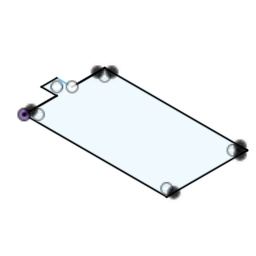
PCB+BOX+V2 (Autodesk Fusion 360 design; units mm, degrees)
Autodesk Fusion 360 part; units mm, degrees
sketch "PCB" plane through (0, 0, 0) normal (0, 0, 1) x (1, 0, 0)
  line L0 (0, 0) -> (92.87, 0)
  line L1 (92.87, 0) -> (92.87, 52.44)
  line L2 (92.87, 52.44) -> (0, 52.44)
  line L3 (0, 0) -> (0, 21.22)
  line L4 (0, 52.44) -> (0, 31.22)
  line L5 (0, 21.22) -> (-10, 21.22)
  line L6 (-10, 21.22) -> (-10, 31.22)
  line L7 (-10, 31.22) -> (0, 31.22)
  line L8 (0, 52.44) -> (0, 31.22)
  line L9 (0, 21.22) -> (0, 0)
  circle A0 centre (-5, 26.22) radius 2.5
  line L10 (0, 52.44) -> (4.6, 52.44)
  line L11 (0, 52.44) -> (0, 47.84)
  circle A1 centre (4.6, 47.84) radius 2
  line L12 (92.87, 52.44) -> (88.27, 52.44)
  line L13 (92.87, 52.44) -> (92.87, 47.84)
  circle A2 centre (88.27, 47.84) radius 2
  line L14 (92.87, 0) -> (92.87, 4.6)
  circle A3 centre (88.27, 4.6) radius 2
  line L15 (0, 0) -> (0, 4.6)
  circle A4 centre (4.6, 4.6) radius 2
  dimension "d8" = 92.87
  dimension "d9" = 52.44
  dimension "d10" = 21.22
  dimension "d11" = 21.22
  dimension "d12" = 10
  dimension "d13" = 5
  dimension "d14" = 4.6
  dimension "d15" = 4.6
  dimension "d16" = 4
  dimension "d17" = 4.6
  dimension "d18" = 4.6
  dimension "d19" = 4
  dimension "d20" = 4.6
  dimension "d21" = 4
  dimension "d22" = 4.6
  dimension "d23" = 4
  constraint horizontal L0
  constraint vertical L1
  constraint horizontal L2
  constraint vertical L8
  constraint coincident L0.start L3.start
  constraint coincident L3.end L8
  constraint horizontal L5
  constraint vertical L6
  constraint horizontal L7
  constraint collinear L8 L9
  constraint perpendicular L4 L10
  constraint perpendicular L2 L11
  constraint perpendicular L1 L12
  constraint perpendicular L12 L13
  constraint perpendicular L2 L14
  constraint perpendicular L0 L15
  measures "d8" distance of L0.start L0.end
  measures "d9" distance of L0.start L2.end
  measures "d10" distance of L0.start L3.end
  measures "d11" distance of L2.end L4.end
  measures "d12" distance of L3.end L5.end
  measures "d13" diameter of A0
  measures "d14" distance of L2.end L10.end
  measures "d15" distance of L2.end L11.end
  measures "d16" diameter of A1
  measures "d17" distance of L1.end L12.end
  measures "d18" distance of L1.end L13.end
  measures "d19" diameter of A2
  measures "d20" distance of L0.end L14.end
  measures "d21" diameter of A3
  measures "d22" distance of L0.start L15.end
  measures "d23" diameter of A4
extrude "Extrude1" add sketch "PCB" along normal blind 1.6 makes body 1
sketch "PCB BOX" plane through (0, 0, 0) normal (0, 0, 1) x (1, 0, 0)
  line L0 (-14.127, 62.44) -> (96.997, 62.44)
  line L1 (102.87, 56.567) -> (102.87, -4.127)
  line L2 (96.997, -10) -> (-14.127, -10)
  line L3 (-20, -4.127) -> (-20, 56.567)
  line L4 (92.87, 52.44) -> (0, 52.44)
  line L5 (92.87, 0) -> (92.87, 52.44)
  line L6 (0, 0) -> (92.87, 0)
  line L7 (-10, 31.22) -> (-10, 21.22)
  line L8 (105.87, 60.44) -> (105.87, -8)
  arc A0 (100.87, -13) -> (105.87, -8) centre (100.87, -8) ccw
  line L9 (100.87, -13) -> (-18, -13)
  arc A1 (-23, -8) -> (-18, -13) centre (-18, -8) ccw
  line L10 (-23, -8) -> (-23, 60.44)
  arc A2 (-18, 65.44) -> (-23, 60.44) centre (-18, 60.44) ccw
  line L11 (-18, 65.44) -> (100.87, 65.44)
  arc A3 (105.87, 60.44) -> (100.87, 65.44) centre (100.87, 60.44) ccw
  circle A4 centre (-18, 60.44) radius 1.45
  arc A5 (-18.75, 57.5353) -> (-15.0953, 61.19) centre (-18, 60.44) ccw
  arc A6 (-18.75, 57.5353) -> (-20, 56.567) centre (-19, 56.567) ccw
  arc A7 (-14.127, 62.44) -> (-15.0953, 61.19) centre (-14.127, 61.44) ccw
  circle A8 centre (-18, -8) radius 1.45
  arc A9 (-15.0953, -8.75) -> (-18.75, -5.0953) centre (-18, -8) ccw
  arc A10 (-20, -4.127) -> (-18.75, -5.0953) centre (-19, -4.127) ccw
  arc A11 (-15.0953, -8.75) -> (-14.127, -10) centre (-14.127, -9) ccw
  circle A12 centre (100.87, 60.44) radius 1.45
  arc A13 (97.9653, 61.19) -> (101.62, 57.5353) centre (100.87, 60.44) ccw
  arc A14 (97.9653, 61.19) -> (96.997, 62.44) centre (96.997, 61.44) ccw
  arc A15 (102.87, 56.567) -> (101.62, 57.5353) centre (101.87, 56.567) ccw
  circle A16 centre (100.87, -8) radius 1.45
  arc A17 (101.62, -5.0953) -> (97.9653, -8.75) centre (100.87, -8) ccw
  arc A18 (96.997, -10) -> (97.9653, -8.75) centre (96.997, -9) ccw
  arc A19 (101.62, -5.0953) -> (102.87, -4.127) centre (101.87, -4.127) ccw
  circle A20 centre (88.27, 47.84) radius 2
  circle A21 centre (-5, 26.22) radius 2.5
  circle A22 centre (88.27, 4.6) radius 2
  circle A23 centre (4.6, 4.6) radius 2
  circle A24 centre (4.6, 47.84) radius 2
  line L12 (92.87, 0) -> (92.87, 52.44)
  line L13 (92.87, 52.44) -> (0, 52.44)
  line L14 (0, 52.44) -> (0, 31.22)
  line L15 (0, 31.22) -> (-10, 31.22)
  line L16 (-10, 31.22) -> (-10, 21.22)
  line L17 (-10, 21.22) -> (0, 21.22)
  line L18 (0, 21.22) -> (0, 0)
  line L19 (0, 0) -> (92.87, 0)
  circle A25 centre (4.6, 47.84) radius 0.775
  circle A26 centre (88.27, 47.84) radius 0.775
  circle A27 centre (4.6, 4.6) radius 0.775
  circle A28 centre (88.27, 4.6) radius 0.775
  circle A29 centre (4.6, 4.6) radius 2.5
  circle A30 centre (4.6, 47.84) radius 2.5
  circle A31 centre (88.27, 47.84) radius 2.5
  circle A32 centre (88.27, 4.6) radius 2.5
  line L20 (7.1, 47.84) -> (7.1, 62.44)
  line L21 (2.1, 62.44) -> (2.1, 47.84)
  line L22 (102.87, 50.34) -> (102, 50.34)
  line L23 (85.77, -10) -> (85.77, 4.6)
  line L24 (90.77, -10) -> (90.77, 4.6)
  line L25 (2.1, -10) -> (2.1, 4.6)
  line L26 (7.1, -10) -> (7.1, 4.6)
  line L27 (85.77, 62.44) -> (85.77, 47.84)
  line L28 (90.77, 62.44) -> (90.77, 47.84)
  circle A33 centre (-18, 60.44) radius 1.125
  circle A34 centre (100.87, 60.44) radius 1.125
  circle A35 centre (-18, -8) radius 1.125
  circle A36 centre (100.87, -8) radius 1.125
  circle A37 centre (-5, 26.22) radius 7.0711
  dimension "d26" = 10
  dimension "d27" = 10
  dimension "d28" = 10
  dimension "d29" = 10
  dimension "d32" = 2.9
  dimension "d33" = 6
  dimension "d34" = 1
  dimension "d35" = 2.9
  dimension "d36" = 6
  dimension "d37" = 1
  dimension "d38" = 2.9
  dimension "d39" = 6
  dimension "d40" = 1
  dimension "d41" = 2.9
  dimension "d42" = 6
  dimension "d43" = 1
  dimension "d53" = 1.55
  dimension "d54" = 1.55
  dimension "d55" = 1.55
  dimension "d56" = 1.55
  dimension "d57" = 5
  dimension "d58" = 5
  dimension "d59" = 5
  dimension "d60" = 5
  dimension "d64" = 2.25
  dimension "d65" = 2.25
  dimension "d66" = 2.25
  dimension "d67" = 2.25
  constraint horizontal L0
  constraint vertical L1
  constraint horizontal L2
  constraint vertical L3
  constraint concentric A4 A5
  constraint tangent L8 A3
  constraint tangent A0 L9
  constraint tangent L8 A0
  constraint tangent L11 A3
  constraint tangent A2 L11
  constraint tangent L10 A2
  constraint tangent L9 A1
  constraint tangent A1 L10
  constraint tangent L3 A6
  constraint tangent A5 A6
  constraint tangent L0 A7
  constraint tangent A5 A7
  constraint equal A6 A7
  constraint concentric A8 A9
  constraint tangent A9 A10
  constraint tangent L3 A10
  constraint tangent A9 A11
  constraint tangent L2 A11
  constraint equal A10 A11
  constraint tangent A13 A14
  constraint tangent L0 A14
  constraint tangent A13 A15
  constraint tangent L1 A15
  constraint equal A14 A15
  constraint concentric A0 A16
  constraint concentric A16 A17
  constraint tangent A17 A18
  constraint tangent L2 A18
  constraint tangent A17 A19
  constraint tangent L1 A19
  constraint equal A18 A19
  constraint concentric A24 A25
  constraint concentric A20 A26
  constraint concentric A23 A27
  constraint concentric A22 A28
  constraint concentric A27 A29
  constraint concentric A24 A30
  constraint concentric A20 A31
  constraint concentric A28 A32
  constraint coincident L0 L20.end
  constraint perpendicular L0 L20
  constraint coincident L0 L21.start
  constraint perpendicular L0 L21
  constraint coincident L1 L22.start
  constraint perpendicular L1 L22
  constraint coincident L2 L23.start
  constraint perpendicular L2 L23
  constraint coincident L2 L24.start
  constraint perpendicular L19 L24
  constraint coincident L2 L25.start
  constraint perpendicular L19 L25
  constraint coincident L2 L26.start
  constraint perpendicular L6 L26
  constraint tangent A29 L25
  constraint tangent A29 L26
  constraint tangent A32 L23
  constraint tangent A32 L24
  constraint tangent A30 L20
  constraint tangent A30 L21
  constraint coincident L0 L27.start
  constraint perpendicular L0 L27
  constraint coincident L0 L28.start
  constraint perpendicular L0 L28
  constraint tangent A31 L27
  constraint tangent A31 L28
  constraint coincident A30 L20.start
  constraint coincident A30 L21.end
  constraint coincident A31 L27.end
  constraint coincident A31 L28.end
  constraint coincident A32 L23.end
  constraint coincident A32 L24.end
  constraint coincident A29 L25.end
  constraint coincident A29 L26.end
  constraint concentric A2 A33
  constraint concentric A13 A34
  constraint concentric A9 A35
  constraint concentric A0 A36
  constraint concentric A21 A37
  constraint coincident L17.end A37
  measures "d26" distance of L0 L4
  measures "d27" distance of L1 L5
  measures "d28" distance of L2 L6
  measures "d29" distance of L3 L7
  measures "d32" diameter of A4
  measures "d33" diameter of A5
  measures "d34" radius of A6
  measures "d35" diameter of A8
  measures "d36" diameter of A9
  measures "d37" radius of A10
  measures "d38" diameter of A12
  measures "d39" diameter of A13
  measures "d40" radius of A14
  measures "d41" diameter of A16
  measures "d42" diameter of A17
  measures "d43" radius of A18
  measures "d53" diameter of A25
  measures "d54" diameter of A26
  measures "d55" diameter of A27
  measures "d56" diameter of A28
  measures "d57" diameter of A29
  measures "d58" diameter of A30
  measures "d59" diameter of A31
  measures "d60" diameter of A32
  measures "d64" diameter of A33
  measures "d65" diameter of A34
  measures "d66" diameter of A35
  measures "d67" diameter of A36
extrude "Extrude2" add sketch "PCB BOX" along normal blind 2 from surface at -8 separate body contours L0 L2 L3 L4 L6 A5 A6 A7 A9 A10 A11 L13 L14 L18 L19 L21 L25 A37 | L0 L4 L13 L20 L21 | L0 L4 L13 L20 L27 | L4 L5 L6 L12 L13 L14 L18 L19 A29 A30 A31 A32 L20 L21 L23 L24 L25 L26 L27 L28 A37 | L4 L13 A30 L20 L21 | L0 L4 L13 L27 L28 | A30 | L0 L1 L2 L4 L5 L6 A13 A14 A15 A17 A18 A19 L12 L13 L19 L24 L28 | L4 L13 A31 L27 L28 | L7 L15 L16 L17 A37 | L15 A37 | A31 | L7 L16 A37 | L17 A37 | L2 L6 L19 L23 L24 | L6 L19 A32 L23 L24 | L6 L19 A29 L25 L26 | L2 L6 L19 L25 L26 | L2 L6 L19 L23 L26 | A32 | A29 | A20 | A21 | A22 | A23 | A24 | A25 | A26 | A27 | A28 makes body 2
extrude "Extrude3" add sketch "PCB BOX" along normal blind 30 from surface at -8 contours L8 A0 L9 A1 L10 A2 L11 A3 | A4 | A8 | A12 | A16 | A33 | A34 | A35 | A36 bodies 2
extrude "Extrude4" cut sketch "PCB BOX" along normal blind 40 from surface at 4 contours A4 | A8 | A12 | A16 | A33 | A34 | A35 | A36 bodies 2
extrude "Extrude5" add sketch "PCB BOX" against normal blind 5 from surface at -1 contours L0 L4 L13 L20 L21 | L4 L13 A30 L20 L21 | L0 L4 L13 L27 L28 | A30 | L4 L13 A31 L27 L28 | A31 | L2 L6 L19 L23 L24 | L6 L19 A32 L23 L24 | L6 L19 A29 L25 L26 | L2 L6 L19 L25 L26 | A32 | A29 | A20 | A22 | A23 | A24 bodies 2
extrude "Extrude6" add sketch "PCB BOX" along normal blind 7 from surface at 30 separate body contours L0 L2 L3 L4 L6 A5 A6 A7 A9 A10 A11 L13 L14 L18 L19 L21 L25 A37 | L0 L4 L13 L20 L21 | L0 L4 L13 L20 L27 | L4 L5 L6 L12 L13 L14 L18 L19 A29 A30 A31 A32 L20 L21 L23 L24 L25 L26 L27 L28 A37 | L4 L13 A30 L20 L21 | L0 L4 L13 L27 L28 | A30 | L0 L1 L2 L4 L5 L6 A13 A14 A15 A17 A18 A19 L12 L13 L19 L24 L28 | L4 L13 A31 L27 L28 | L7 L15 L16 L17 A37 | L15 A37 | A31 | L7 L16 A37 | L17 A37 | L2 L6 L19 L23 L24 | L6 L19 A32 L23 L24 | L6 L19 A29 L25 L26 | L2 L6 L19 L25 L26 | L2 L6 L19 L23 L26 | A32 | A29 | L8 A0 L9 A1 L10 A2 L11 A3 | A4 | A8 | A12 | A16 | A20 | A21 | A22 | A23 | A24 | A25 | A26 | A27 | A28 makes body 3
extrude "Extrude7" cut sketch "PCB BOX" along normal blind 40 from surface at 10 contours L7 L15 L16 L17 A37 | L15 A37 | L7 L16 A37 | L17 A37 | A21 bodies 3
extrude "Extrude8" cut sketch "PCB BOX" against normal blind 20 from surface at -2 contours L7 L15 L16 L17 A37 | L15 A37 | L7 L16 A37 | L17 A37 | A21 bodies 2
hidden bodies 3
named bodies: "PCB", "PCB BOX", "PCB BOX LID"
